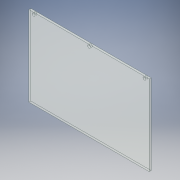
# Autodesk Inventor part: Perspex shield
Saved by Autodesk Inventor 2019 (Build 230136000, 136)
## iProperties
Created: 2021-03-05
Part Number: Perspex shield
Material: Glass
Document SubType Name: Modeling
Designer: User
Density: 2.18 g/cm^3
Appearance: Clear
Author: User
Autodesk Inventor part; units mm, degrees
ref_plane "YZ Plane" through (0, 0, 0) normal (1, 0, 0) x (0, 1, 0)
ref_plane "XZ Plane" through (0, 0, 0) normal (0, 1, 0) x (-1, 0, 0)
ref_plane "XY Plane" through (0, 0, 0) normal (0, 0, 1) x (1, 0, 0)
sketch "Sketch1" plane through (0, 0, 0) normal (0, 0, 1) x (1, 0, 0)
  line L0 (-157.1429, 200) -> (142.8571, 200)
  line L1 (142.8571, 200) -> (142.8571, 0)
  line L2 (142.8571, 0) -> (-157.1429, 0)
  line L3 (-157.1429, 0) -> (-157.1429, 200)
  point P0 (0, 0)
  dimension "d0" = 200
  dimension "d1" = 300
  dimension "d2" = 142.8571
  dimension "d3" = 200
  constraints: 8 end point, 2 parallel, 1 horizontal, 1 perpendicular
  measures "d0" distance between parallel lines of L2 L0
  measures "d1" distance between parallel lines of L3 L1
  measures "d2" distance from line of point (0, 0) L1
  measures "d3" distance from line of point (0, 0) L0
extrude "Extrusion1" add sketch "Sketch1" along normal blind 5
sketch "Sketch3" plane through (0, 0, 5) normal (0, 0, 1) x (1, 0, 0)
  circle A0 centre (130.8571, 195) radius 3.5
  circle A1 centre (-145.1429, 195) radius 3.5
  circle A2 centre (-7.1429, 195) radius 3.5
  line L0 (142.8571, 0) -> (142.8571, 200) projected
  line L1 (-157.1429, 200) -> (-157.1429, 0) projected
  line L2 (142.8571, 200) -> (-157.1429, 200) projected
  point P0 (0, 0)
  dimension "d6" = 7
  dimension "d7" = 7
  dimension "d8" = 7
  dimension "d9" = 12
  dimension "d10" = 12
  dimension "d11" = 150
  dimension "d12" = 5
  dimension "d13" = 5
  dimension "d14" = 5
  constraints: 3 centre point
  measures "d6" diameter of A0
  measures "d7" diameter of A1
  measures "d8" diameter of A2
  measures "d9" distance from line of A0.centre L0
  measures "d10" distance from line of L1 A1.centre
  measures "d11" distance from line of L1 A2.centre
  measures "d12" distance from line of A0.centre L2
  measures "d13" distance from line of L2 A2.centre
  measures "d14" distance from line of L2 A1.centre
extrude "Extrusion2" cut sketch "Sketch3" against normal blind 10
body "Solid1"
